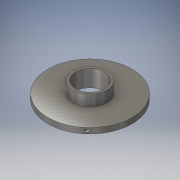
# Autodesk Inventor part: Top1
Saved by Autodesk Inventor 2016 (Build 200138000, 138)
## iProperties
Created: 2015-11-28
Part Number: Top1
Material: Generic
Document SubType Name: Modeling
Designer: Javier
Density: 1 g/cm^3
Appearance: Diamond Plate
Author: Javier
Autodesk Inventor part; units mm, degrees
ref_plane "YZ Plane" through (0, 0, 0) normal (1, 0, 0) x (0, 1, 0)
ref_plane "XZ Plane" through (0, 0, 0) normal (0, 1, 0) x (-1, 0, 0)
ref_plane "XY Plane" through (0, 0, 0) normal (0, 0, 1) x (1, 0, 0)
sketch "Sketch1" plane through (0, 0, 0) normal (0, 1, 0) x (-1, 0, 0)
  circle A0 centre (0, 0) radius 190.5
  dimension "d0" = 381
  constraints: 1 centre point, 1 coincident
  measures "d0" diameter of A0
extrude "Extrusion1" add sketch "Sketch1" along normal blind 25.4
sketch "Sketch2" plane through (0, 25.4, 0) normal (0, 1, 0) x (1, 0, 0)
  circle A0 centre (0, 0) radius 76.2
  dimension "d3" = 152.4
  constraints: 1 centre point, 1 coincident
  measures "d3" diameter of A0
extrude "Extrusion2" add sketch "Sketch2" along normal blind 50.8
sketch "Sketch3" plane through (0, 0, 0) normal (0, 1, 0) x (-1, 0, 0)
  circle A0 centre (0, 0) radius 66.04
  dimension "d6" = 132.08
  constraints: 1 centre point, 1 coincident
  measures "d6" diameter of A0
extrude "Extrusion3" cut sketch "Sketch3" along normal up to next
sketch "Sketch10" plane through (0, 0, 0) normal (0, 0, 1) x (1, 0, 0)
  line L0 (25.4, 12.7) -> (-25.4, 12.7) projected
  circle A0 centre (127, 12.7) radius 6.35
  circle A1 centre (-127, 12.7) radius 6.35
  point P0 (0, 0)
  dimension "d37" = 12.7
  dimension "d38" = 12.7
  dimension "d41" = 254
  constraints: 2 centre point
  measures "d37" diameter of A0
  measures "d38" diameter of A1
  measures "d41" distance of A0.centre A1.centre
extrude "Extrusion10" cut sketch "Sketch10" along normal mid plane 508
body "Solid1"
